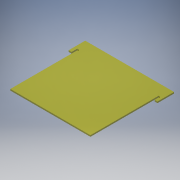
# Autodesk Inventor part: door
Saved by Autodesk Inventor 2019 (Build 230136000, 136)
## iProperties
Created: 2015-05-02
Part Number: door
Material: Generic
Document SubType Name: Modeling
Designer: cruiser
Density: 1 g/cm^3
Appearance: Clear - Yellow
Author: cruiser
Autodesk Inventor part; units mm, degrees
ref_plane "YZ Plane" through (0, 0, 0) normal (1, 0, 0) x (0, 1, 0)
ref_plane "XZ Plane" through (0, 0, 0) normal (0, 1, 0) x (-1, 0, 0)
ref_plane "XY Plane" through (0, 0, 0) normal (0, 0, 1) x (1, 0, 0)
sketch "Sketch1" plane through (0, 0, 0) normal (0, 0, 1) x (1, 0, 0)
  line L0 (90.5, -89.56) -> (-90.5, -89.56)
  line L1 (-90.5, -89.56) -> (-90.5, 89.56)
  line L2 (-90.5, 89.56) -> (90.5, 89.56)
  line L3 (90.5, 89.56) -> (90.5, -89.56)
  line L4 (90.5, -89.56) -> (-90.5, 89.56) construction
  line L5 (-90.5, -89.56) -> (90.5, 89.56) construction
  line L6 (90.5, 89.56) -> (93.65, 89.56)
  line L7 (93.65, 89.56) -> (93.65, 64.56)
  line L8 (93.65, 64.56) -> (90.5, 64.56)
  line L9 (90.5, 64.56) -> (90.5, 89.56)
  line L10 (0, 0) -> (0, 89.56)
  line L11 (-90.5, 89.56) -> (-93.65, 89.56)
  line L12 (-93.65, 89.56) -> (-93.65, 64.56)
  line L13 (-93.65, 64.56) -> (-90.5, 64.56)
  line L14 (-90.5, 64.56) -> (-90.5, 89.56)
  dimension "d0" = 179.12
  dimension "d1" = 181
  dimension "d2" = 3.15
  dimension "d3" = 25
  constraints: 30 end point, 4 parallel, 3 midpoint, 3 symmetric about line, 2 horizontal, 2 perpendicular
  measures "d0" distance of L0.end L1.end
  measures "d1" distance of L0.start L0.end
  measures "d2" distance of L7.end L8.end
  measures "d3" distance of L6.end L7.end
extrude "Extrusion1" add sketch "Sketch1" along normal blind 3.15
sketch "Sketch2" plane through (0, 0, 3.15) normal (0, 0, 1) x (1, 0, 0)
  line L0 (93.65, 89.56) -> (-93.65, 89.56) projected
  line L1 (-93.65, 89.56) -> (-100.37, 89.56)
  line L2 (-100.37, 89.56) -> (-100.37, 52.06)
  line L3 (-100.37, 52.06) -> (-93.65, 52.06)
  line L4 (-93.65, 52.06) -> (-93.65, 89.56)
  line L5 (0, 89.56) -> (0, 0)
  line L6 (93.65, 89.56) -> (93.65, 64.56)
  line L7 (93.65, 89.56) -> (100.37, 89.56)
  line L8 (100.37, 89.56) -> (100.37, 52.06)
  line L9 (100.37, 52.06) -> (93.65, 52.06)
  line L10 (93.65, 52.06) -> (93.65, 89.56)
  point P0 (-93.65, 64.56)
  dimension "d6" = 6.72
  dimension "d7" = 12.5
  constraints: 20 end point, 3 parallel, 3 symmetric about line, 1 horizontal, 1 midpoint, 1 perpendicular
  measures "d6" distance of L3.end L2.end
  measures "d7" distance from line of point (-93.65, 64.56) L3
extrude "Extrusion2" add sketch "Sketch2" against normal blind 3.15
sketch "Sketch5" plane through (0, 0, 3.15) normal (0, 0, 1) x (1, 0, 0)
  line L0 (-93.65, 64.56) -> (-90.5, 64.56) projected
  circle A0 centre (-93.65, 64.56) radius 0.25
  circle A1 centre (-90.5, 64.56) radius 0.25
  line L1 (0, 0) -> (0, 89.56)
  line L2 (100.37, 89.56) -> (-100.37, 89.56) projected
  circle A2 centre (93.65, 64.56) radius 0.25
  circle A3 centre (90.5, 64.56) radius 0.25
  dimension "d19" = 0.5
  dimension "d20" = 0.5
  constraints: 4 centre point, 2 end point, 2 symmetric about line, 1 coincident, 1 midpoint, 2 other
  measures "d19" diameter of A0
  measures "d20" diameter of A1
extrude "Extrusion5" cut sketch "Sketch5" against normal up to next
fillet "Fillet1" radius 0.25 2 edges at (-93.65, 52.06, 1.575) (93.65, 52.06, 1.575)
sketch "Sketch3" plane through (-90.5, -89.56, 0) normal (0, -1, 0) x (1, 0, 0)
  line L0 (0, 0) -> (181, 0) projected
  line L1 (0, 3.15) -> (181, 3.15) projected
  line L2 (113.65, 3.15) -> (142.85, 3.15)
  line L3 (142.85, 3.15) -> (142.85, 0)
  line L4 (142.85, 0) -> (113.65, 0)
  line L5 (113.65, 0) -> (113.65, 3.15)
  line L6 (128.25, 3.15) -> (128.25, 0)
  point P0 (90.5, 0)
  dimension "d10" = 29.2
  dimension "d11" = 37.75
  constraints: 10 end point, 2 midpoint, 2 parallel, 2 point on line, 1 horizontal, 1 perpendicular
  measures "d10" distance between parallel lines of L5 L3
  measures "d11" distance from line of point (90.5, 0) L6
sketch "Sketch4" plane through (0, 0, 3.15) normal (0, 0, 1) x (1, 0, 0)
  line L0 (-90.5, -89.56) -> (23.15, -89.56) projected
  line L1 (52.35, -110.16) -> (23.15, -110.16) projected
  circle A0 centre (47.75, -105.16) radius 1.575
  line L2 (0, 0) -> (0, -89.56)
  dimension "d14" = 5
  dimension "d15" = 47.75
  dimension "d16" = 3.15
  constraints: 2 end point, 1 centre point, 1 perpendicular, 1 point on line
  measures "d14" distance from line of L1 A0.centre
  measures "d15" distance from line of A0.centre L2
  measures "d16" diameter of A0
equation "\"d2\" = t_window"
equation "\"t_door\" = t_window"
equation "\"d8\" = t_door"
equation "\"d11\" = protection_slot_offset"
equation "\"d16\" = m3_diameter"
equation "\"wood_thickness\" = 6.72"
equation "\"m3_diameter\" = 3.15"
equation "\"m5_diameter\" = 5.25"
equation "\"stepper_screw_space\" = 35"
equation "\"stepper_shaft_diameter\" = 5"
equation "\"stepper_body_diameter\" = 28"
equation "\"laser_body_diameter\" = 12"
equation "\"thick_acrylic\" = 5.88"
equation "\"carrier_y\" = 181"
equation "\"carrier_z\" = 233.04"
equation "\"carrier_z2\" = 283.04"
equation "\"window_z\" = 185"
equation "\"window_slot\" = 25"
equation "\"reservoir_x\" = 151"
equation "\"reservoir_y\" = 151"
equation "\"thin_acrylic\" = 3.15"
equation "\"linear_bearing_spacing\" = 207"
equation "\"linear_bearing_z\" = 304.8"
equation "\"threaded_rod_z\" = 203.2"
equation "\"motor_spacing\" = 287"
equation "\"tray_boarder\" = 15"
equation "\"tray_x\" = 151"
equation "\"tray_y\" = 181"
equation "\"brass_insert_drill\" = 4"
equation "\"brass_keep_out\" = 8"
equation "\"tape_keep_out\" = 2"
equation "\"tape_thickness\" = 2"
equation "\"crane_x\" = 244.56"
equation "\"z_min_from_center\" = 72.28"
equation "\"printer_z\" = 289"
equation "\"frame_tilt\" = 0"
equation "\"lcd_x\" = 72"
equation "\"lcd_y\" = 25"
equation "\"clear_acrylic\" = 3.15"
equation "\"laser_y\" = 33"
equation "\"laser_y_offset\" = 19.4"
equation "\"laser_diameter\" = 12"
equation "\"laser_z\" = 33"
equation "\"subframe_y_offset\" = 27.5"
equation "\"frame_top_z\" = 295"
equation "\"frame_y\" = 68.44"
equation "\"frame_bottom_z\" = 225"
equation "\"t_frame\" = 6.72"
equation "\"frame_border\" = 39.5"
equation "\"t_carrier\" = 6.72"
equation "\"t_tray\" = 3.15"
equation "\"tray_border\" = 15"
equation "\"t_wall\" = 5.88"
equation "\"galvo_frame_z\" = 65"
equation "\"galvo_frame_x\" = 66"
equation "\"t_galvo_frame\" = 6.72"
equation "\"galvo_frame_y_offset\" = 27.5"
equation "\"m4_diameter\" = 4.2"
equation "\"window_y\" = 49.56"
equation "\"t_window\" = 3.15"
equation "\"laser_x\" = 62"
equation "\"drawer_z\" = 206.72"
equation "\"drawer_x\" = 181"
equation "\"drawer_y\" = 49.56"
equation "\"frame_foot_z\" = 49.5"
equation "\"drawer_z_from_bottom\" = 25"
equation "\"end_stop_offset_x\" = 83"
equation "\"t_crane\" = 6.72"
equation "\"end_stop_spacing\" = 19"
equation "\"thumb_nut_offset_y\" = 11.72"
equation "\"thumb_nut_diameter\" = 7"
equation "\"frame_foot_extension\" = 6"
equation "\"m5_brass_insert_drill\" = 6.7"
equation "\"m3_brass_insert_drill\" = 4"
equation "\"door_sensor\" = 35"
equation "\"protection_slot_offset\" = 37.75"
equation "\"protection_slot\" = 30.2"
equation "\"protection_slot_length\" = 20.6"
equation "\"m3_main_nut_width\" = 5.7"
equation "\"m3_main_extra\" = 1"
equation "\"m3_main_length\" = 14"
equation "\"m3_main_nut_thickness\" = 2.5"
equation "\"al1_thickness\" = 1.5875"
equation "\"bed_t\" = 1.5875"
equation "\"bed_fold_x\" = 15"
equation "\"bed_gap\" = 0.3"
equation "\"bed_y2\" = 45.96"
equation "\"m5_press_nut_drill\" = 6.35"
equation "\"asym_key\" = 0"
equation "\"small_round\" = 2"
equation "\"drawer_foot_mount\" = 18"
equation "\"inner_tray_x\" = 145"
equation "\"t_tape\" = 3"
equation "\"inner_tray_radius\" = 24"
equation "\"t_inner_tray\" = 5.88"
equation "\"inner_tray_border\" = 5"
equation "\"inner_tray_y\" = 145"
equation "\"bottom_clear_border\" = 5"
equation "\"t_bottom_clear\" = 3.15"
equation "\"laser_screw_spacing_y\" = 16"
body "Solid1"
